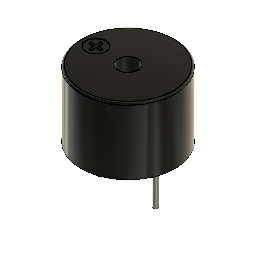
Buzzer (Autodesk Fusion 360 design; units mm, degrees)
Autodesk Fusion 360 part; units mm, degrees
sketch "Sketch1" plane through (0, 0, 0) normal (0, 0, 1) x (1, 0, 0)
  circle A0 centre (0, 0) radius 6
  circle A1 centre (0, 0) radius 1.25
  line L0 (-6, 0.0236) -> (6, 0.0236) construction
  line L1 (-6, 0.0236) -> (-3.5, 0.0236) construction
  line L2 (6, 0.0236) -> (3.5, 0.0236) construction
  circle A2 centre (3.5, 0.0236) radius 0.3
  circle A3 centre (-3.5, 0.0236) radius 0.3
  dimension "d1" = 12
  dimension "d2" = 2.5
  dimension "d3" = 2.5
  dimension "d5" = 2.5
  dimension "d6" = 0.6
  dimension "d7" = 0.6
  constraint coincident A0.centre A1.centre
  constraint concentric A0 A1
  constraint coincident A0 L0.start
  constraint coincident A0 L0.end
  constraint horizontal L0
  constraint parallel L0 L1
  constraint parallel L0 L2
  constraint coincident L2.end A2.centre
  constraint coincident L1.end A3.centre
  measures "d1" diameter of A0
  measures "d2" diameter of A1
  measures "d3" distance of L0.start L1.end
  measures "d5" distance of L0.end L2.end
  measures "d6" diameter of A2
  measures "d7" diameter of A3
extrude "Extrude1" add sketch "Sketch1" along normal blind 8.5 contours A0 | A1 | A2 | A3
sketch "Sketch2" plane through (0, 0, 8.5) normal (0, 0, 1) x (-1, 0, 0)
  circle A0 centre (0, 0) radius 6
  circle A1 centre (0, 0) radius 1.25
  circle A2 centre (4.0974, 0) radius 1.25
  line L0 (3.9724, 0.75) -> (4.2224, 0.75)
  line L1 (4.2224, 0.75) -> (4.2224, -0.75)
  line L2 (4.2224, -0.75) -> (3.9724, -0.75)
  line L3 (3.9724, -0.75) -> (3.9724, 0.75)
  line L4 (3.9724, 0.75) -> (4.2224, -0.75) construction
  line L5 (4.2224, 0.75) -> (3.9724, -0.75) construction
  line L6 (4.8474, -0.125) -> (3.3474, -0.125)
  line L7 (4.8474, 0.125) -> (4.8474, -0.125)
  line L8 (3.3474, 0.125) -> (4.8474, 0.125)
  line L9 (3.3474, -0.125) -> (3.3474, 0.125)
  point P0 (4.0974, 0)
  dimension "d14" = 2.5
  dimension "d15" = 1.5
  dimension "d16" = 0.25
  dimension "d18" = 90
  constraint perpendicular L0 L1
  constraint parallel L0 L2
  constraint parallel L1 L3
  constraint horizontal L0
  constraint coincident L4 P0
  constraint coincident L5 P0
  constraint coincident P0 A2.centre
  measures "d14" diameter of A2
  measures "d15" distance of L0.end L1.end
  measures "d16" distance of L1.end L2.end
extrude "Extrude4" cut sketch "Sketch2" against normal blind 0.1 contours A2
extrude "Extrude2" cut sketch "Sketch2" against normal blind 3 contours A1
extrude "Extrude3" add sketch "Sketch1" against normal blind 5.5 contours A2 | A3
fillet "Fillet1" radius 0.25 1 edges at (-5.594, -2.1697, 8.5)
